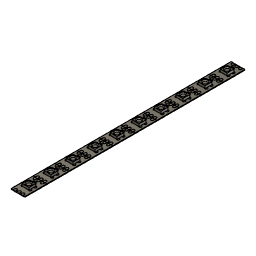
LED_Strip (Autodesk Fusion 360 design; units mm, degrees)
Autodesk Fusion 360 part; units mm, degrees
sketch "Sketch1" plane through (0, 0, 0) normal (0, 1, 0) x (1, 0, 0)
  line L0 (5, 8) -> (-5, 8)
  line L1 (-5, 8) -> (-5, -8)
  line L2 (-5, -8) -> (5, -8)
  line L3 (5, -8) -> (5, 8)
  line L4 (5, 8) -> (-5, -8) construction
  line L5 (-5, 8) -> (5, -8) construction
  line L6 (2.5, 2.5) -> (-2.5, 2.5)
  line L7 (-2.5, 2.5) -> (-2.5, -2.5)
  line L8 (-2.5, -2.5) -> (2.5, -2.5)
  line L9 (2.5, -2.5) -> (2.5, 2.5)
  line L10 (2.5, 2.5) -> (-2.5, -2.5) construction
  line L11 (-2.5, 2.5) -> (2.5, -2.5) construction
  circle A0 centre (2.7, -1.8) radius 0.9
  line L12 (0, 8) -> (0, 7.5894)
  line L13 (0, 7.5894) -> (0, -8) construction
  line L14 (5, 0) -> (-5, 0) construction
  circle A1 centre (2.7, 1.8) radius 0.9
  circle A2 centre (-2.7, -1.8) radius 0.9
  circle A3 centre (-2.7, 1.8) radius 0.9
  line L15 (-0.9, 6) -> (0.9, 6)
  line L16 (0.9, 6) -> (0.9, 10)
  line L17 (0.9, 10) -> (-0.9, 10)
  line L18 (-0.9, 10) -> (-0.9, 6)
  line L19 (-0.9, 6) -> (0.9, 10) construction
  line L20 (0.9, 6) -> (-0.9, 10) construction
  line L21 (-1.8, 10) -> (-3.6, 10)
  line L22 (-3.6, 10) -> (-3.6, 6)
  line L23 (-3.6, 6) -> (-1.8, 6)
  line L24 (-1.8, 6) -> (-1.8, 10)
  line L25 (3.6, 10) -> (1.8, 10)
  line L26 (1.8, 10) -> (1.8, 6)
  line L27 (1.8, 6) -> (3.6, 6)
  line L28 (3.6, 6) -> (3.6, 10)
  line L29 (1, 3.5) -> (-1, 3.5)
  line L30 (-1, 3.5) -> (-1, 4.5)
  line L31 (-1, 4.5) -> (1, 4.5)
  line L32 (1, 4.5) -> (1, 3.5)
  line L33 (1, 3.5) -> (-1, 4.5) construction
  line L34 (-1, 3.5) -> (1, 4.5) construction
  line L35 (-1.8, -10) -> (-3.6, -10)
  line L36 (-3.6, -10) -> (-3.6, -6)
  line L37 (-1.8, -6) -> (-1.8, -10)
  line L38 (-3.6, -6) -> (-1.8, -6)
  line L39 (-0.9, -10) -> (-0.9, -6)
  line L40 (0.9, -10) -> (-0.9, -10)
  line L41 (0.9, -6) -> (0.9, -10)
  line L42 (-0.9, -6) -> (0.9, -6)
  line L43 (1.8, -6) -> (3.6, -6)
  line L44 (3.6, -6) -> (3.6, -10)
  line L45 (1.8, -10) -> (1.8, -6)
  line L46 (3.6, -10) -> (1.8, -10)
  point P0 (0, 8)
  point P1 (0, 4)
  dimension "d1" = 10
  dimension "d2" = 16
  dimension "d3" = 5
  dimension "d4" = 5
  dimension "d5" = 1.8
  dimension "d6" = 1.8
  dimension "d7" = 4
  dimension "d10" = 2.7
  dimension "d11" = 0
  dimension "d12" = 2
  dimension "d13" = 1
  dimension "d14" = 1
  constraint horizontal L0
  constraint perpendicular L0 L1
  constraint parallel L0 L2
  constraint parallel L1 L3
  constraint coincident L4 origin
  constraint coincident L5 origin
  constraint horizontal L6
  constraint perpendicular L6 L7
  constraint parallel L6 L8
  constraint parallel L7 L9
  constraint coincident L10 origin
  constraint coincident L11 origin
  constraint midpoint L0 P0
  constraint perpendicular L0 L12
  constraint midpoint L2 L13.end
  constraint perpendicular L2 L13
  constraint midpoint L3 L14.start
  constraint midpoint L1 L14.end
  constraint symmetric A0 L14 A1
  constraint symmetric A0 L13 A2
  constraint symmetric L13 A1 A3
  constraint horizontal L15
  constraint perpendicular L15 L16
  constraint parallel L15 L17
  constraint parallel L16 L18
  constraint coincident L19 P0
  constraint coincident L20 P0
  constraint coincident P0 L12.start
  constraint horizontal L29
  constraint perpendicular L29 L30
  constraint parallel L29 L31
  constraint parallel L30 L32
  constraint coincident L33 P1
  constraint coincident L34 P1
  constraint coincident L13 P1
  constraint symmetric L14 L15.start L39.end
  constraint symmetric L14 L15.end L41.start
  constraint symmetric L14 L16.end L40.start
  constraint symmetric L14 L17.end L39.start
  constraint symmetric L14 L21.start L35.start
  constraint symmetric L14 L21.end L35.end
  constraint symmetric L14 L22.end L36.end
  constraint symmetric L14 L23.end L37.start
  constraint symmetric L14 L25.start L44.end
  constraint symmetric L14 L25.end L45.start
  constraint symmetric L14 L26.end L43.start
  constraint symmetric L14 L27.end L43.end
  measures "d1" distance of L1.end L2.end
  measures "d2" distance of L0.end L1.end
  measures "d3" distance of L7.end L8.end
  measures "d4" distance of L6.end L7.end
  measures "d5" diameter of A0
  measures "d6" distance of L16.end L17.end
  measures "d7" distance of L15.end L16.end
  measures "d12" distance of L30.end L31.end
  measures "d13" distance of L29.end L30.end
  measures "d14" distance of L6 L29
extrude "Extrude1" add sketch "Sketch1" against normal blind 0.45 contours L0 L1 L2 L3 L15 L16 L18 L22 L23 L24 L26 L27 L28 L36 L37 L38 L39 L41 L42 L43 L44 L45 | L0 L26 L27 L28 | L2 L43 L44 L45 | L0 L15 L16 L18 | L2 L39 L41 L42 | L0 L22 L23 L24 | L2 L36 L37 L38 | L6 L9 A1 | L6 L9 A1 | L6 L7 L8 L9 A0 A1 A2 A3 | L6 L7 A3 | L6 L7 A3 | L8 L9 A0 | L8 L9 A0 | L7 L8 A2 | L7 L8 A2 | L29 L30 L31 L32 makes body 1
extrude "Extrude2" add sketch "Sketch1" along normal blind 1 separate body contours L29 L30 L31 L32 makes body 2
extrude "Extrude3" add sketch "Sketch1" along normal blind 1.75 contours L6 L9 A1 | L6 L7 L8 L9 A0 A1 A2 A3 | L6 L7 A3 | L8 L9 A0 | L7 L8 A2 picked at (2.4573, 1.4615) picked at (-2.4571, 1.4615) picked at (2.4573, -1.4615) picked at (-2.4571, -1.4615) bodies 1
extrude "Extrude4" cut sketch "Sketch1" against normal blind 0.1 contours L0 L26 L27 L28 | L2 L43 L44 L45 | L0 L15 L16 L18 | L2 L39 L41 L42 | L0 L22 L23 L24 | L2 L36 L37 L38 | L6 L9 A1 | L6 L7 A3 | L8 L9 A0 | L7 L8 A2 picked at (2.8098, 1.4616) picked at (-2.8103, 1.4618) picked at (2.8098, -1.4616) picked at (-2.8103, -1.4618) bodies 1
fillet "Fillet1" radius 0.9 12 edges at (-1.8, -0.05, 6) (-3.6, -0.05, 6) (-0.9, -0.05, 6) (0.9, -0.05, 6) (1.8, -0.05, 6) (3.6, -0.05, 6) (-0.9, -0.05, -6) (1.8, -0.05, -6) (0.9, -0.05, -6) (-1.8, -0.05, -6) (-3.6, -0.05, -6) (3.6, -0.05, -6) on bodies 1
fillet "Fillet2" radius 0.3 2 edges at (-1, 1, -4) (1, 1, -4) on bodies 2
fillet "Fillet3" radius 0.2 10 edges at (-1, 0.35, -3.5) (-0.9121, 0.9121, -3.5) (0, 1, -3.5) (0.9121, 0.9121, -3.5) (1, 0.35, -3.5) (-1, 0.35, -4.5) (-0.9121, 0.9121, -4.5) (0, 1, -4.5) (0.9121, 0.9121, -4.5) (1, 0.35, -4.5) on bodies 2
sketch "Sketch2" plane through (0, 1.75, 0) normal (0, 1, 0) x (-1, 0, 0)
  line L0 (-2.5, 2.5) -> (-2.5, -2.5)
  line L1 (-2.5, -2.5) -> (2.5, -2.5)
  line L2 (2.5, -2.5) -> (2.5, 2.5)
  line L3 (2.5, 2.5) -> (-2.5, 2.5)
  line L4 (2.5, -1.6515) -> (1.6515, -2.5)
  line L5 (2.5, -1.6515) -> (3.7, -1.6515) construction
  line L6 (-2.5, -2.5) -> (2.5, -2.5)
  circle A0 centre (0, 0) radius 2
  dimension "d29" = 135
  dimension "d30" = 1.2
  dimension "d31" = 4
  constraint horizontal L5
  constraint coincident L2 L4.start
  constraint coincident L4.end L6
  constraint coincident A0.centre origin
  measures "d29" angle of L4 L5
  measures "d30" distance of L4.start L4.end
  measures "d31" diameter of A0
extrude "Extrude5" cut sketch "Sketch2" against normal blind 0.3 contours L1 L2 L4 L6 bodies 1
extrude "Extrude6" cut sketch "Sketch2" against normal blind 0.6 contours A0 bodies 1
chamfer "Chamfer1" distance 0.6 angle 45 1 edges at (1.8647, 1.15, 0.7232) on bodies 1
combine "Combine1" operation add target body 1 tool bodies 2
pattern_linear "R-Pattern2" count 10 spacing 16 along (0, 0, 1) of bodies 1 makes body 3 at (-1.6667, -0.45, 18.6667) makes body 4 at (-1.6667, -0.45, 34.6667) makes body 5 at (-1.6667, -0.45, 50.6667) makes body 6 at (-1.6667, -0.45, 66.6667) makes body 7 at (-1.6667, -0.45, 82.6667) makes body 8 at (-1.6667, -0.45, 98.6667) makes body 9 at (-1.6667, -0.45, 114.6667) makes body 10 at (-1.6667, -0.45, 130.6667) makes body 11 at (-1.6667, -0.45, 146.6667)
equation "d10 = 0.9 mm + d6"
equation "d24 = d6 / 2"
equation "depth = -0.6 mm"
equation "d36 = -depth"
equation "numLEDs = 10"
equation "d43 = numLEDs"
equation "d45 = d2"
